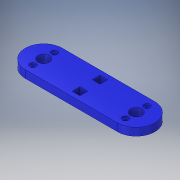
# Autodesk Inventor part: Middle_leg_a
Saved by Autodesk Inventor 2017 (Build 210142000, 142)
## iProperties
Created: 2016-06-08
Part Number: Middle_leg_a
Material: Generic
Document SubType Name: Modeling
Designer: alex-
Density: 1 g/cm^3
Appearance: Blue - Wall Paint - Glossy
Author: alex-
Autodesk Inventor part; units mm, degrees
ref_plane "YZ Plane" through (0, 0, 0) normal (1, 0, 0) x (0, 1, 0)
ref_plane "XZ Plane" through (0, 0, 0) normal (0, 1, 0) x (-1, 0, 0)
ref_plane "XY Plane" through (0, 0, 0) normal (0, 0, 1) x (1, 0, 0)
sketch "Sketch1" plane through (0, 0, 0) normal (0, 1, 0) x (-1, 0, 0)
  circle A0 centre (30, 0) radius 12
  circle A1 centre (-30, 0) radius 12
  line L0 (30, 12) -> (-30, 12)
  line L1 (30, -12) -> (-30, -12)
  circle A2 centre (30, 0) radius 3.75
  circle A3 centre (-30, 0) radius 3.75
  line L2 (58.8, 0) -> (-58.8, 0) projected
  line L3 (2.5, -9) -> (-2.5, -9)
  line L4 (-2.5, -9) -> (-2.5, -4)
  line L5 (-2.5, -4) -> (2.5, -4)
  line L6 (2.5, -4) -> (2.5, -9)
  line L7 (2.5, 9) -> (-2.5, 9)
  line L8 (-2.5, 9) -> (-2.5, 4)
  line L9 (-2.5, 4) -> (2.5, 4)
  line L10 (2.5, 4) -> (2.5, 9)
  circle A4 centre (30, -7) radius 1
  circle A5 centre (30, 7) radius 1
  circle A6 centre (-30, -7) radius 1
  circle A7 centre (-30, 7) radius 1
  point P0 (0, 0)
  point P1 (0, 12)
  point P2 (0, -9)
  point P3 (0, 9)
  dimension "d5" = 60
  dimension "d6" = 24
  dimension "d7" = 7.5
  dimension "d12" = 5
  dimension "d13" = 5
  dimension "d14" = 4
  dimension "d17" = 2
  dimension "d18" = 7
  dimension "d19" = 7
  constraints: 20 end point, 8 centre point, 6 vertical alignment, 5 equal radius, 5 symmetric about line, 4 horizontal alignment, 4 point on circle, 3 parallel, 2 coincident, 2 horizontal, 2 midpoint, 2 tangent, 1 perpendicular
  measures "d5" distance of A1.centre A0.centre
  measures "d6" diameter of A0
  measures "d7" diameter of A2
  measures "d12" distance of L5.end L3.start
  measures "d13" distance of L3.start L3.end
  measures "d14" distance between parallel lines of L2 L5
  measures "d17" diameter of A4
  measures "d18" distance of A0.centre A4.centre
  measures "d19" distance of A0.centre A5.centre
extrude "Extrusion5" add sketch "Sketch1" along normal blind 5 contours L2 A2 A0 | A0 L2 A2 | A0 L2 A1 L0 | L1 A1 L2 A0 | A1 L2 A3 | A1 L2 A3
sketch "Sketch3" plane through (0, 5, 0) normal (0, 1, 0) x (1, 0, 0)
  circle A0 centre (-30, 7) radius 2
  circle A1 centre (-30, -7) radius 2
  circle A2 centre (30, 7) radius 2
  circle A3 centre (30, -7) radius 2
  circle A4 centre (-30, 7) radius 1 projected
  circle A5 centre (-30, -7) radius 1 projected
  circle A6 centre (30, 7) radius 1 projected
  circle A7 centre (30, -7) radius 1 projected
  point P0 (0, 0)
  dimension "d22" = 4
  constraints: 4 centre point, 4 concentric, 3 equal radius
  measures "d22" diameter of A0
extrude "Extrusion6" cut sketch "Sketch3" against normal blind 1
equation "\"d6\" = sa_diameter"
equation "\"d12\" = b_mat_thickness"
equation "\"d13\" = b_mat_thickness"
equation "\"d14\" = 0.8 * b_mat_thickness"
equation "\"d20\" = b_mat_thickness"
equation "\"sa_diameter\" = 24"
equation "\"b_mat_thickness\" = 5"
body "Solid3"
